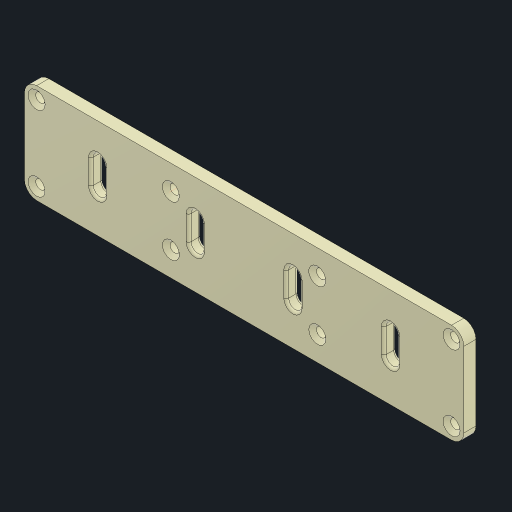
# Autodesk Inventor part: SKÅDIS Pegboard Back
Saved by Autodesk Inventor 2024 (Build 280153000, 153)
## iProperties
Created: 2024-02-08
Part Number: SKÅDIS Pegboard Back
Material: 일반
Document SubType Name: Modeling
Designer: KBU
Density: 1 g/cm^3
Appearance: 기본값
Author: KBU
Autodesk Inventor part; units mm, degrees
ref_plane "XZ Plane" through (0, 0, 0) normal (0, 1, 0) x (-1, 0, 0)
sketch "스케치1" plane through (0, 0, 0) normal (0, 0, 1) x (1, 0, 0)
  line L0 (-90, -20.375) -> (90, -20.375)
  line L1 (90, -20.375) -> (90, 20.375)
  line L2 (90, 20.375) -> (-90, 20.375)
  line L3 (-90, 20.375) -> (-90, -20.375)
  line L4 (-90, -20.375) -> (90, 20.375) construction
  line L5 (90, -20.375) -> (-90, 20.375) construction
  point P0 (0, 0)
  dimension "d0" = 180
  dimension "d1" = 40.75
  constraints: 12 end point, 2 midpoint, 2 parallel, 1 horizontal, 1 perpendicular
  measures "d0" distance of L1.end L2.end
  measures "d1" distance of L2.end L0.start
extrude "돌출1" add sketch "스케치1" along normal blind 5
fillet "모깎기1" radius 5 4 edges at (90, -20.375, 2.5) (-90, -20.375, 2.5) (-90, 20.375, 2.5) (90, 20.375, 2.5)
sketch "스케치2" plane through (0, 0, 5) normal (0, 0, 1) x (1, 0, 0)
  line L0 (90, 20.375) -> (-90, 20.375) projected
  line L1 (-90, 20.375) -> (-90, -20.375) projected
  line L2 (-90, -20.375) -> (90, -20.375) projected
  line L3 (-60, -4.375) -> (-60, 5.625) construction
  line L4 (-57.25, -4.375) -> (-57.25, 5.625)
  line L5 (-62.75, 5.625) -> (-62.75, -4.375)
  arc A0 (-62.75, -4.375) -> (-57.25, -4.375) centre (-60, -4.375) ccw
  arc A1 (-57.25, 5.625) -> (-62.75, 5.625) centre (-60, 5.625) ccw
  line L6 (-20, -4.375) -> (-20, 5.625) construction
  line L7 (-17.25, -4.375) -> (-17.25, 5.625)
  line L8 (-22.75, 5.625) -> (-22.75, -4.375)
  arc A2 (-22.75, -4.375) -> (-17.25, -4.375) centre (-20, -4.375) ccw
  arc A3 (-17.25, 5.625) -> (-22.75, 5.625) centre (-20, 5.625) ccw
  line L9 (20, -4.375) -> (20, 5.625) construction
  line L10 (22.75, -4.375) -> (22.75, 5.625)
  line L11 (17.25, 5.625) -> (17.25, -4.375)
  arc A4 (17.25, -4.375) -> (22.75, -4.375) centre (20, -4.375) ccw
  arc A5 (22.75, 5.625) -> (17.25, 5.625) centre (20, 5.625) ccw
  line L12 (60, -4.375) -> (60, 5.625) construction
  line L13 (62.75, -4.375) -> (62.75, 5.625)
  line L14 (57.25, 5.625) -> (57.25, -4.375)
  arc A6 (57.25, -4.375) -> (62.75, -4.375) centre (60, -4.375) ccw
  arc A7 (62.75, 5.625) -> (57.25, 5.625) centre (60, 5.625) ccw
  circle A8 centre (-30, 10.375) radius 3.5
  circle A9 centre (-30, 10.375) radius 1.95
  line L15 (-104.0692, 0) -> (93.9823, 0)
  line L16 (0, 34.3163) -> (0, -28.4805)
  circle A10 centre (-85, 15.375) radius 1.95
  circle A11 centre (-85, 15.375) radius 3.5
  circle A12 centre (-30, -10.375) radius 3.5
  circle A13 centre (-30, -10.375) radius 1.95
  circle A14 centre (-85, -15.375) radius 1.95
  circle A15 centre (-85, -15.375) radius 3.5
  circle A16 centre (30, 10.375) radius 3.5
  circle A17 centre (30, 10.375) radius 1.95
  circle A18 centre (85, 15.375) radius 1.95
  circle A19 centre (85, 15.375) radius 3.5
  circle A20 centre (85, -15.375) radius 3.5
  circle A21 centre (85, -15.375) radius 1.95
  circle A22 centre (30, -10.375) radius 3.5
  circle A23 centre (30, -10.375) radius 1.95
  point P0 (0, 0)
  point P1 (-60, 0.625)
  point P2 (-60, -7.125)
  point P3 (-60, 8.375)
  point P4 (-20, 0.625)
  point P5 (-20, -7.125)
  point P6 (-20, 8.375)
  point P7 (20, 0.625)
  point P8 (20, -7.125)
  point P9 (20, 8.375)
  point P10 (60, 0.625)
  point P11 (60, -7.125)
  point P12 (60, 8.375)
  dimension "d4" = 5.5
  dimension "d5" = 15.5
  dimension "d6" = 30
  dimension "d7" = 13.25
  dimension "d10" = 40
  dimension "d19" = 3.9
  dimension "d20" = 7
  dimension "d22" = 30
  dimension "d23" = 10
  dimension "d25" = 7
  dimension "d26" = 3.9
  dimension "d27" = 5
  dimension "d28" = 5
  constraints: 36 end point, 24 centre point, 18 point on circle, 12 symmetric about line, 8 coincident, 4 tangent, 3 horizontal, 3 vertical, 1 midpoint, 1 parallel, 54 other
  measures "d4" distance between parallel lines of L4 L5
  measures "d5" distance of point (-60, -7.125) point (-60, 8.375)
  measures "d6" distance from line of L1 point (-60, 0.625)
  measures "d7" distance from line of point (-60, -7.125) L2
  measures "d10" distance of L4.start L7.start
  measures "d19" diameter of A9
  measures "d20" diameter of A8
  measures "d22" horizontal distance of point (0, 0) A8.centre
  measures "d23" distance from line of L0 A8.centre
  measures "d25" diameter of A11
  measures "d26" diameter of A10
  measures "d27" distance from line of L0 A11.centre
  measures "d28" distance from line of L1 A11.centre
extrude "돌출2" cut sketch "스케치2" against normal through all contours L15 L8 A3 L7 | L7 A2 L8 L15 | L15 L4 A0 L5 | L5 A1 L4 L15 | A4 L11 L15 L10 | L15 L11 A5 L10 | A6 L14 L15 L13 | L15 L14 A7 L13 | A9 | A10 | A13 | A14 | A17 | A18 | A21 | A23
extrude "돌출3" cut sketch "스케치2" against normal blind 1.561 contours A8 | A11 | A12 | A15 | A16 | A19 | A20 | A22
fillet "모깎기3" radius 1 32 edges at (-62.75, 0.625, 0) (-60, -7.125, 0) (-57.25, 0.625, 0) (-60, 8.375, 0) (-57.25, 0.625, 5) (-60, -7.125, 5) (-62.75, 0.625, 5) (-60, 8.375, 5) (-22.75, 0.625, 0) (-20, -7.125, 0) (-17.25, 0.625, 0) (-20, 8.375, 0) (-17.25, 0.625, 5) (-20, -7.125, 5) (-22.75, 0.625, 5) (-20, 8.375, 5) (17.25, 0.625, 0) (20, -7.125, 0) (22.75, 0.625, 0) (20, 8.375, 0) (22.75, 0.625, 5) (20, -7.125, 5) (17.25, 0.625, 5) (20, 8.375, 5) (57.25, 0.625, 0) (60, -7.125, 0) (62.75, 0.625, 0) (60, 8.375, 0) (62.75, 0.625, 5) (60, -7.125, 5) (57.25, 0.625, 5) (60, 8.375, 5)
chamfer "모따기1" distance 0.1 angle 45 8 edges at (-86.95, 15.375, 0) (-86.95, -15.375, 0) (-31.95, 10.375, 0) (-31.95, -10.375, 0) (28.05, -10.375, 0) (28.05, 10.375, 0) (83.05, 15.375, 0) (83.05, -15.375, 0)
ref_plane "작업 평면1" through (-85, -15.375, 0) normal (-1, 0, 0) x (0, 0, 1)
sketch "스케치3" plane through (-85, -15.375, 0) normal (-1, 0, 0) x (0, 0, 1)
  line L0 (3.439, 32.7) -> (0.1, 32.7) projected
  line L1 (5, 34.25) -> (5, 27.25) projected
  line L2 (3.4388, 32.7) -> (5, 34.25)
  line L3 (3.439, 32.7) -> (3.4388, 32.7)
  line L4 (5, 30.75) -> (0, 30.75) projected
  line L5 (5, 30.75) -> (6.9247, 30.75)
  line L6 (3.439, 34.25) -> (3.439, 27.25) projected
  line L7 (5, 34.25) -> (3.439, 34.25)
  line L8 (3.439, 34.25) -> (3.439, 32.7)
  point P0 (0, 15.375)
  point P1 (3.439, 32.7002)
  dimension "d39" = 2.2
  dimension "d40" = 0.0003
  constraints: 10 end point, 3 horizontal, 1 collinear, 1 point on line
  measures "d39" distance of L2.start L1.start
  measures "d40" distance of L0.start L2.start
revolve "회전1" add sketch "스케치3" angle 360 about axis through (-85, 15.375, 5) along (0, 0, 1) contours L2 L6 L7
mirror "미러1" about plane through (0, 0, 0) normal (0, 1, 0) of "회전1"
mirror "미러2" about plane through (0, 0, 0) normal (1, 0, 0) of "회전1", "미러1"
ref_plane "작업 평면2" through (-30, 0, 0) normal (1, 0, 0) x (0, 1, 0)
sketch "스케치4" plane through (-30, 0, 0) normal (1, 0, 0) x (0, 1, 0)
  line L0 (6.875, 5) -> (13.875, 5) projected
  line L1 (6.875, 5) -> (8.4295, 3.439)
  line L2 (6.875, 3.439) -> (13.875, 3.439) projected
  line L3 (6.875, 3.439) -> (6.875, 5)
  line L4 (6.875, 5) -> (6.875, 3.439) projected
  line L5 (6.875, 3.439) -> (8.4295, 3.439)
  line L6 (12.325, 0.1) -> (8.425, 0.1) projected
  line L7 (10.375, 0.1) -> (10.375, 6.4669)
  point P0 (0, 0)
  constraints: 8 end point, 1 collinear, 1 midpoint, 1 perpendicular, 1 point on line, 1 vertical
revolve "회전2" add sketch "스케치4" angle 360 about axis through (-30, 10.375, 0.1) along (0, 0, 1) contours L1 L2 L3
mirror "미러3" about plane through (0, 0, 0) normal (0, 1, 0) of "회전2"
mirror "미러4" about plane through (0, 0, 0) normal (1, 0, 0) of "회전2", "미러3"
